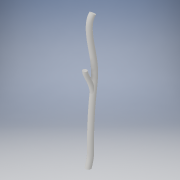
# Autodesk Inventor part: stick_0
Saved by Autodesk Inventor 2018 (Build 220112000, 112)
## iProperties
Created: 2018-10-22
Part Number: stick_0
Material: Generic
Document SubType Name: Modeling
Designer: Gage
Density: 1 g/cm^3
Appearance: Default
Author: Gage
Autodesk Inventor part; units mm, degrees
ref_plane "YZ Plane" through (0, 0, 0) normal (1, 0, 0) x (0, 1, 0)
ref_plane "XY Plane" through (0, 0, 0) normal (0, 0, 1) x (1, 0, 0)
sketch "Sketch1" plane through (0, 0, 0) normal (0, 1, 0) x (-1, 0, 0)
  circle A0 centre (0, 0) radius 31.75
  dimension "d0" = 63.5
  constraints: 1 centre point, 1 coincident
  measures "d0" diameter of A0
sketch "Sketch2" plane through (0, 0, 0) normal (1, 0, 0) x (0, 1, 0)
  spline S0 degree 4 poles (0, 0) (161.2772, -47.8235) (85.8066, -13.4528) (966.837, -42.269) (1032.9883, -139.0121) (1515.1235, 61.0576) (1625.2831, -56.2794) knots 0 0 0 0 0 0.365984 0.541691 1 1 1 1 1
  point P0 (131.9755, -28.9407)
  point P1 (271.8806, -28.9408)
  point P2 (736.4269, -56.2793)
  point P3 (1010.7652, -78.2264)
  point P4 (1332.6555, -28.9408)
  constraints: 7 other
sweep "Sweep1" add profiles "Sketch1" path "Sketch2"
sketch "Sketch3" plane through (0, 0, 0) normal (1, 0, 0) x (0, 1, 0)
  spline S0 degree 3 poles (736.4217, -56.2787) (882.9348, -63.143) (1008.2153, 46.8352) (1060.5781, 39.1639) knots 0 0 0 0 1 1 1 1
  point P0 (0, 0)
  point P1 (1625.2831, -56.2794)
  point P2 (910.4588, -18.5737)
  point P3 (1016.6971, 29.926)
  constraints: 6 other
ref_plane "Work Plane1" through (0, 736.4217, -56.2787) normal (0, 1, 0) x (-1, 0, 0)
sketch "Sketch4" plane through (0, 736.4217, -56.2787) normal (0, 1, 0) x (-1, 0, 0)
  circle A0 centre (0, -0.0006) radius 25.4
  point P0 (0, 56.2787)
  dimension "d5" = 50.8
  constraints: 1 centre point, 1 coincident
  measures "d5" diameter of A0
sweep "Sweep2" add profiles "Sketch4" path "Sketch3"
body "Solid1"
